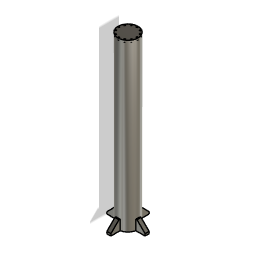
base_link (Autodesk Fusion 360 design; units mm, degrees)
Autodesk Fusion 360 part; units mm, degrees
note: some values were not read from the file. Set by a fixed rule: which sketch regions a step uses.
sketch "Boceto1" plane through (0, 0, 0) normal (0, 1, 0) x (1, 0, 0)
  circle A0 centre (0, 0) radius 100
  circle A1 centre (0, 0) radius 90
  line L0 (0, 0) -> (0, 90)
  line L1 (0, 0) -> (90, 0)
  line L2 (0, 0) -> (0, -90)
  line L3 (0, 0) -> (-90, 0)
  line L4 (0, 0) -> (77.9423, 45)
  line L5 (0, 0) -> (82.5, 0) construction
  line L6 (0, 0) -> (45, 77.9423)
  line L7 (0, 0) -> (82.5, 0) construction
  line L8 (0, 0) -> (-45, 77.9423)
  line L9 (0, 0) -> (82.5, 0) construction
  line L10 (0, 0) -> (-77.9423, 45)
  line L11 (0, 0) -> (82.5, 0) construction
  line L12 (0, 0) -> (-90, 0)
  line L13 (0, 0) -> (-77.9423, -45)
  line L14 (0, 0) -> (-45, -77.9423)
  line L15 (0, 0) -> (-82.5, 0) construction
  line L16 (0, 0) -> (0, -90)
  line L17 (0, 0) -> (45, -77.9423)
  line L18 (0, 0) -> (77.9423, -45)
  line L19 (0, 0) -> (82.5, 0) construction
  circle A2 centre (0, 90) radius 7.5
  circle A3 centre (-45, 77.9423) radius 7.5
  circle A4 centre (-77.9423, 45) radius 7.5
  circle A5 centre (-90, 0) radius 7.5
  circle A6 centre (-77.9423, -45) radius 7.5
  circle A7 centre (-45, -77.9423) radius 7.5
  circle A8 centre (0, -90) radius 7.5
  circle A9 centre (45, -77.9423) radius 7.5
  circle A10 centre (77.9423, -45) radius 7.5
  circle A11 centre (90, 0) radius 7.5
  circle A12 centre (77.9423, 45) radius 7.5
  circle A13 centre (45, 77.9423) radius 7.5
  dimension "d1" = 200
  dimension "d14" = 180
  dimension "d16" = 30
  dimension "d17" = 60
  dimension "d18" = 120
  dimension "d19" = 150
  dimension "d20" = 30
  dimension "d21" = 60
  dimension "d22" = 30
  dimension "d23" = 30
  dimension "d24" = 15
  dimension "d25" = 15
  dimension "d26" = 15
  dimension "d27" = 15
  dimension "d28" = 15
  dimension "d29" = 15
  dimension "d30" = 15
  dimension "d31" = 15
  dimension "d32" = 15
  dimension "d33" = 15
  dimension "d34" = 15
  dimension "d35" = 15
  constraint coincident A0.centre A1.centre
  constraint coincident A1 L0.end
  constraint vertical L0
  constraint coincident A1 L1.end
  constraint perpendicular L0 L1
  constraint coincident A1 L2.end
  constraint perpendicular L1 L2
  constraint coincident A1 L3.end
  constraint perpendicular L2 L3
  constraint horizontal L5
  constraint horizontal L7
  constraint horizontal L9
  constraint horizontal L11
  constraint horizontal L15
  constraint coincident A1 L14.end
  constraint coincident A1 L17.end
  constraint horizontal L19
  constraint coincident L0.end A2.centre
  constraint coincident A1 L8.end
  constraint coincident A1 L10.end
  constraint coincident A1 L13.end
  constraint coincident A1 L18.end
  constraint coincident A1 L4.end
  constraint coincident A1 L6.end
  constraint coincident L8.end A3.centre
  constraint coincident L10.end A4.centre
  constraint coincident L3.end L12.end
  constraint coincident L13.end A6.centre
  constraint coincident L14.end A7.centre
  constraint coincident L2.end L16.end
  constraint coincident L17.end A9.centre
  constraint coincident L18.end A10.centre
  constraint coincident L1.end A11.centre
  constraint coincident L4.end A12.centre
  constraint coincident L6.end A13.centre
  measures "d1" diameter of A0
  measures "d14" diameter of A1
  measures "d16" angle of L4 L5
  measures "d17" angle of L6 L7
  measures "d18" angle of L8 L9
  measures "d19" angle of L10 L11
  measures "d20" angle of L12 L13
  measures "d21" angle of L14 L15
  measures "d22" angle of L16 L17
  measures "d23" angle of L18 L19
  measures "d24" diameter of A2
  measures "d25" diameter of A3
  measures "d26" diameter of A4
  measures "d27" diameter of A5
  measures "d28" diameter of A6
  measures "d29" diameter of A7
  measures "d30" diameter of A8
  measures "d31" diameter of A9
  measures "d32" diameter of A10
  measures "d33" diameter of A11
  measures "d34" diameter of A12
  measures "d35" diameter of A13
extrude "Extruir1" add sketch "Boceto1" along normal blind 1650 contours A0 | A1 L1 L4 A11 A12 | A1 L1 L18 A10 A11 | A1 L0 L8 A2 A3 | A1 L2 L16 L17 A8 A9 | A1 L3 L12 L13 A5 A6 | A1 L4 L6 A12 A13 | A1 L0 L6 A2 A13 | A1 L8 L10 A3 A4 | A1 L3 L10 L12 A4 A5 | A1 L13 L14 A6 A7 | A1 L2 L14 L16 A7 A8 | A1 L17 L18 A9 A10
extrude "Extruir2" add sketch "Boceto1" along normal blind 1630 contours A1 L1 A11 | A1 A11 | A1 L1 A11 | A1 L4 A12 | A1 A12 | A1 A10 | A1 L18 A10 | A1 L4 A12 | A1 L18 A10 | A1 L0 A2 | A1 L0 A2 | A1 L2 L16 A8 | A1 L2 L16 A8 | A1 L3 L12 A5 | A1 L3 L12 A5 | A1 L6 A13 | A1 L6 A13 | A1 L8 A3 | A1 L8 A3 | A1 L10 A4 | A1 L10 A4 | A1 L13 A6 | A1 L13 A6 | A1 L14 A7 | A1 L14 A7 | A1 L17 A9 | A1 L17 A9 | A1 A2 | A1 A8 | A1 A5 | A1 A13 | A1 A3 | A1 A4 | A1 A6 | A1 A7 | A1 A9
sketch "Boceto2" plane through (0, 0, 0) normal (1, 0, 0) x (0, 0, -1)
  line L0 (70, 0) -> (70, 100)
  line L1 (70, 100) -> (110, 100)
  line L2 (110, 100) -> (190, 20)
  line L3 (190, 20) -> (190, 0)
  line L4 (190, 0) -> (70, 0)
  line L5 (0, 0) -> (0, 40)
  line L6 (-110, 100) -> (-190, 20)
  line L7 (-70, 100) -> (-110, 100)
  line L8 (-70, 0) -> (-70, 100)
  line L9 (-190, 0) -> (-70, 0)
  line L10 (-190, 20) -> (-190, 0)
  line L11 (100, 0) -> (-100, 0)
  dimension "d40" = 40
  dimension "d43" = 20
  dimension "d44" = 120
  dimension "d45" = 100
  constraint vertical L0
  constraint perpendicular L0 L1
  constraint parallel L0 L3
  constraint perpendicular L0 L4
  constraint coincident L5.start origin
  constraint vertical L5
  constraint symmetric L0.start L5 L8.start
  constraint symmetric L0.end L5 L7.start
  constraint symmetric L1.end L5 L6.start
  constraint symmetric L2.end L5 L6.end
  constraint symmetric L3.end L5 L9.start
  measures "d40" distance of L0 L1.end
  measures "d43" distance of L2.end L4
  measures "d44" distance of L0 L3.end
  measures "d45" distance of L0.end L11
extrude "Extruir3" add sketch "Boceto2" along normal mid plane 40
sketch "Boceto3" plane through (0, 0, 0) normal (0, 0, 1) x (1, 0, 0)
  line L0 (-100, 0) -> (-100, 100)
  line L1 (-100, 100) -> (-110, 100)
  line L2 (-100, 0) -> (-190, 0)
  line L3 (-190, 0) -> (-190, 20)
  line L4 (-190, 20) -> (-110, 100)
  line L5 (-100, 100) -> (-70, 100)
  line L6 (-70, 100) -> (-70, 0)
  line L7 (-70, 0) -> (-100, 0)
  line L8 (0, 0) -> (0, 105.8881)
  line L9 (100, 100) -> (70, 100)
  line L10 (70, 100) -> (70, 0)
  line L11 (70, 0) -> (100, 0)
  line L12 (100, 0) -> (190, 0)
  line L13 (190, 0) -> (190, 20)
  line L14 (190, 20) -> (110, 100)
  line L15 (100, 100) -> (110, 100)
  dimension "d46" = 100
  dimension "d47" = 90
  constraint vertical L0
  constraint perpendicular L0 L1
  constraint perpendicular L0 L2
  constraint perpendicular L2 L3
  constraint perpendicular L0 L5
  constraint perpendicular L5 L6
  constraint perpendicular L0 L7
  constraint coincident L8.start origin
  constraint perpendicular L7 L8
  constraint symmetric L0.start L8 L11.end
  constraint symmetric L0.end L8 L9.start
  constraint symmetric L1.end L8 L14.end
  constraint symmetric L2.end L8 L12.end
  constraint symmetric L3.end L8 L13.end
  constraint symmetric L5.end L8 L9.end
  constraint symmetric L6.end L8 L10.end
  measures "d46" distance of L0.start L0.end
  measures "d47" distance of L0.start L2.end
extrude "Extruir4" add sketch "Boceto3" along normal mid plane 40
move_body "Move1" bodies 1 to x (1, 0, 0) y (0, 0, 1) z (0, -1, 0) at (0, 0, 0)
